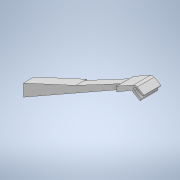
# Autodesk Inventor part: grip - C1-1
Saved by Autodesk Inventor 2020 (Build 240168000, 168)
## iProperties
Created: 2021-05-09
Part Number: grip - C1-1
Material: Generic
Document SubType Name: Modeling
Designer: Hengameh
Density: 1 g/cm^3
Appearance: Default
Author: Hengameh
Autodesk Inventor part; units mm, degrees
ref_plane "YZ Plane" through (0, 0, 0) normal (1, 0, 0) x (0, 1, 0)
ref_plane "XZ Plane" through (0, 0, 0) normal (0, 1, 0) x (-1, 0, 0)
ref_plane "XY Plane" through (0, 0, 0) normal (0, 0, 1) x (1, 0, 0)
sketch "Sketch1" plane through (0, 0, 0) normal (0, 0, 1) x (1, 0, 0)
  line L0 (459.0035, 284.2249) -> (458.9968, 260.6799)
  line L1 (531.739, 304.0541) -> (458.9968, 260.6799)
  arc A0 (531.739, 304.0541) -> (538.4376, 297.9317) centre (549.0074, 316.2218) ccw
  line L2 (538.4376, 297.9317) -> (569.6147, 279.9315)
  line L3 (569.6147, 279.9315) -> (575.6772, 290.432)
  line L4 (575.6772, 290.432) -> (544.4999, 308.4321)
  arc A1 (553.4999, 324.0206) -> (544.4999, 308.4321) centre (548.9999, 316.2263) ccw
  line L5 (553.4999, 324.0206) -> (584.6772, 306.0204)
  line L6 (584.6772, 306.0204) -> (588.2396, 312.1908)
  line L7 (588.2396, 312.1908) -> (557.067, 330.191)
  arc A2 (557.067, 330.191) -> (539.0042, 328.8755) centre (549.0048, 316.2262) ccw
  line L8 (459.0035, 284.2249) -> (539.0042, 328.8755)
  line L9 (0, 0) -> (459.0039, 260.6839)
  line L10 (459.0039, 284.2249) -> (459.0039, 260.6839)
  line L11 (459.0039, 284.2249) -> (248.0021, 171.9727)
  line L12 (248.0021, 171.9727) -> (0, 57.1249)
  line L13 (0, 57.1249) -> (0, 0)
  line L14 (459.0035, 284.2249) -> (539.0042, 328.8755)
  arc A3 (557.067, 330.191) -> (539.0042, 328.8755) centre (549.0048, 316.2266) ccw
  line L15 (459.0035, 284.2249) -> (248.0021, 171.9727)
  line L16 (0, 57.1249) -> (0, 0)
  line L17 (0, 0) -> (569.6147, 0) construction
  line L18 (569.6147, 0) -> (569.6147, 279.9315) construction
  point P0 (459.0039, 260.6841)
  point P1 (459.0035, 284.2247)
  dimension "SUR_H" = 57.1249
  dimension "GRIP_H" = 330.191
  dimension "PIN_TH" = 7.1249
  dimension "PIN_TH2" = 12.1249
  dimension "PIN_R" = 9
  dimension "OUT_PIN_R" = 16.125
  dimension "PIN_TO_SUR" = 548.9999
  dimension "d7" = 588.2396
  dimension "d8" = 279.9315
  dimension "d9" = 29.594
  dimension "d10" = 24.849
  dimension "d11" = 28.013
  dimension "d12" = 30.806
  dimension "d13" = 248.0021
  dimension "d14" = 211.0014
  dimension "d15" = 171.9727
  dimension "d16" = 284.2249
  dimension "d17" = 316.2264
  dimension "d18" = 60
  dimension "d19" = 149.996
  dimension "d20" = 312.1908
  dimension "d21" = 90
  dimension "d22" = 90
  dimension "d23" = 90
  dimension "d24" = 21.1247
  dimension "d25" = 17.2609
  dimension "d26" = 12.1723
  dimension "d27" = 10.5672
  dimension "d28" = 12.6491
  dimension "d29" = 9.9957
  dimension "d30" = 18.2947
  constraints: 38 end point, 8 point on circle, 4 centre point, 1 coincident, 1 collinear, 1 horizontal, 1 perpendicular, 1 point on line
  measures "SUR_H" distance of L12.end L9.start
  measures "GRIP_H" vertical distance of point (0, 0) L7.end
  measures "PIN_TH" distance of L5.end L6.end
  measures "PIN_TH2" distance of L2.end L3.end
  measures "PIN_R" radius of A1
  measures "OUT_PIN_R" radius of A2
  measures "PIN_TO_SUR" horizontal distance of point (0, 0) A1.centre
  measures "d7" horizontal distance of L6.end point (0, 0)
  measures "d8" vertical distance of L2.end point (0, 0)
  measures "d9" angle of L17 L9
  measures "d10" angle of L17 L12
  measures "d11" angle of L17 L11
  measures "d12" angle of L17 L1
  measures "d13" horizontal distance of L11.end L12.end
  measures "d14" horizontal distance of L0.start L11.end
  measures "d15" vertical distance of point (0, 0) L11.end
  measures "d16" vertical distance of point (0, 0) L0.start
  measures "d17" vertical distance of point (0, 0) A1.centre
  measures "d18" angle of L17 L3
  measures "d19" angle of L17 L7
  measures "d20" distance from line of L17 L6.end
  measures "d21" angle of L6 L5
  measures "d22" angle of L3 L4
  measures "d23" angle of L3 L2
  measures "d24" radius of A0
  measures "d25" horizontal distance of A1.centre L1.start
  measures "d26" vertical distance of L1.start A1.centre
  measures "d27" horizontal distance of A3.centre L2.start
  measures "d28" vertical distance of A1.centre L8.end
  measures "d29" horizontal distance of A1.centre L8.end
  measures "d30" vertical distance of A1.centre L2.start
extrude "Extrusion1" add sketch "Sketch1" along normal mid plane 80 contours L8 A2 L7 L6 L5 A1 L4 L3 L2 A0 L1 L10 | L0 L9 L13 L12 L11
sketch "Sketch2" plane through (0, 0, 40) normal (0, 0, 1) x (1, 0, 0)
  line L0 (458.9968, 260.6799) -> (458.9982, 284.2219)
  line L1 (539.0042, 328.8755) -> (459.0035, 284.2249) projected
  line L2 (459.0035, 284.2247) -> (248.0021, 171.9727) projected
  line L3 (0, 57.1249) -> (0, 0) projected
  line L4 (248.0021, 171.9727) -> (0, 57.1249)
  line L5 (0, 57.1249) -> (0, 0)
  line L6 (0, 0) -> (458.9968, 260.6799)
  line L7 (459.0039, 260.6841) -> (531.739, 304.0541) projected
  point P0 (458.9982, 284.2219)
  dimension "d33" = 59.19
  constraints: 8 end point, 1 collinear, 1 point on line
  measures "d33" angle of L7 L0
extrude "Extrusion2" cut sketch "Sketch2" against normal blind 20
mirror "Mirror1" about plane through (0, 0, 0) normal (0, 0, 1) of "Extrusion2"
sketch "Sketch3" plane through (0, 0, -20) normal (0, 0, -1) x (-1, 0, 0)
  line L0 (0, 57.1249) -> (-248.0021, 171.9727) projected
  line L1 (-248.0021, 171.9727) -> (-248.0021, 140.8488)
  line L2 (-458.9968, 260.6799) -> (0, 0) projected
  line L3 (0, 0) -> (0, 57.1249)
  constraints: 4 end point, 2 vertical, 1 point on line
extrude "Extrusion3" add sketch "Sketch3" along normal blind 10
body "Solid1"
